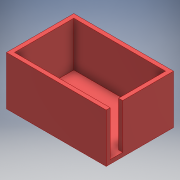
# Autodesk Inventor part: box
Saved by Autodesk Inventor 2018 (Build 220112000, 112)
## iProperties
Created: 2018-01-24
Part Number: box
Material: Generic
Document SubType Name: Modeling
Designer: mokuz
Density: 1 g/cm^3
Appearance: Smooth - Red
Author: mokuz
Autodesk Inventor part; units mm, degrees
ref_plane "YZ Plane" through (0, 0, 0) normal (1, 0, 0) x (0, 1, 0)
ref_plane "XZ Plane" through (0, 0, 0) normal (0, 1, 0) x (-1, 0, 0)
ref_plane "XY Plane" through (0, 0, 0) normal (0, 0, 1) x (1, 0, 0)
sketch "Sketch1" plane through (0, 0, 0) normal (0, 0, 1) x (1, 0, 0)
  line L0 (0, 0) -> (400, 0)
  line L1 (400, 0) -> (400, 270)
  line L2 (400, 270) -> (0, 270)
  line L3 (0, 270) -> (0, 0)
  dimension "d0" = 400
  dimension "d1" = 270
  constraints: 8 end point, 2 parallel, 1 horizontal, 1 perpendicular
  measures "d0" distance of L2.end L1.end
  measures "d1" distance of L1.end L0.end
extrude "Extrusion1" add sketch "Sketch1" along normal blind 16
sketch "Sketch2" plane through (0, 0, 16) normal (0, 0, 1) x (1, 0, 0)
  line L0 (0, 0) -> (400, 0) projected
  line L1 (400, 0) -> (400, 270) projected
  line L2 (400, 270) -> (0, 270) projected
  line L3 (0, 270) -> (0, 0) projected
  line L4 (16, 16) -> (384, 16)
  line L5 (384, 16) -> (384, 254)
  line L6 (384, 254) -> (16, 254)
  line L7 (16, 254) -> (16, 16)
  dimension "d4" = 16
  dimension "d5" = 16
  dimension "d6" = 16
  dimension "d7" = 16
  constraints: 8 end point, 2 parallel, 1 horizontal, 1 perpendicular
  measures "d4" distance between parallel lines of L3 L7
  measures "d5" distance between parallel lines of L1 L5
  measures "d6" distance between parallel lines of L2 L6
  measures "d7" distance between parallel lines of L4 L0
extrude "Extrusion2" add sketch "Sketch2" along normal blind 180
sketch "Sketch3" plane through (0, 0, 196) normal (0, 0, 1) x (1, 0, 0)
  line L0 (16, 254) -> (16, 16) projected
  line L1 (16, 16) -> (384, 16) projected
  line L2 (384, 16) -> (384, 254) projected
  line L3 (384, 254) -> (16, 254) projected
  line L4 (384, 254) -> (384, 16) projected
  line L5 (400, 0) -> (400, 270) projected
  line L6 (384, 16) -> (400, 16)
  line L7 (400, 16) -> (400, 66)
  line L8 (400, 66) -> (384, 66)
  line L9 (384, 66) -> (384, 16)
  point P0 (0, 0)
  dimension "d10" = 50
  constraints: 8 end point, 2 parallel, 1 horizontal, 1 perpendicular, 1 point on line
  measures "d10" distance of L7.end L6.end
extrude "Extrusion3" cut sketch "Sketch3" against normal blind 180 contours L2 L8 L5 L6
body "Solid1"
